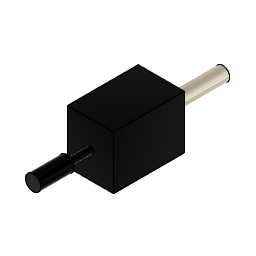
Large Solenoid Triggerable v13 (Autodesk Fusion 360 archive; units mm, degrees)
design "Self-retaining (two-way) Electromagnet DC 12V Push-pull Solenoid"
Autodesk Fusion 360 part; units mm, degrees
sketch "Sketch1" plane through (0, 0, 0) normal (0, 1, 0) x (1, 0, 0)
  line L0 (7.45, -8.575) -> (-7.45, -8.575)
  line L1 (-7.45, -8.575) -> (-7.45, 8.575)
  line L2 (-7.45, 8.575) -> (7.45, 8.575)
  line L3 (7.45, 8.575) -> (7.45, -8.575)
  line L4 (7.45, -8.575) -> (-7.45, 8.575) construction
  line L5 (-7.45, -8.575) -> (7.45, 8.575) construction
  circle A0 centre (0, 0) radius 1
  circle A1 centre (0, 0) radius 1.1
  dimension "d1" = 14.9
  dimension "d2" = 17.15
  dimension "d5" = 2.2
  dimension "d6" = 2
  constraint horizontal L0
  constraint perpendicular L0 L1
  constraint parallel L0 L2
  constraint parallel L1 L3
  constraint coincident L4 A0.centre
  constraint coincident L5 A0.centre
  constraint coincident A0.centre A1.centre
  measures "d1" distance of L1.end L2.end
  measures "d2" distance of L0.end L1.end
  measures "d5" diameter of A1
  measures "d6" diameter of A0
extrude "Extrude1" add sketch "Sketch1" along normal mid plane 22.85 contours L0 L1 L2 L3 makes body 1
extrude "Extrude2" add sketch "Sketch1" along normal blind 42.7 and the other way blind 18.5 from surface at -11.425 separate body contours A0 makes body 2
sketch "Sketch2" plane through (0, -29.925, 0) normal (0, -1, 0) x (1, 0, 0)
  circle A0 centre (0, 0) radius 1
  circle A1 centre (0, 0) radius 2.5
  dimension "d11" = 5
  constraint concentric A0 A1
  measures "d11" diameter of A1
extrude "Extrude3" add sketch "Sketch2" against normal blind 10.78 bodies 1 2
sketch "Sketch3" plane through (0, 31.275, 0) normal (0, 1, 0) x (-1, 0, 0)
  circle A0 centre (0, 0) radius 1
  circle A1 centre (0, 0) radius 2.25
  dimension "d15" = 4.5
  constraint concentric A0 A1
  measures "d15" diameter of A1
extrude "Extrude4" add sketch "Sketch3" against normal blind 14.5 bodies 2
copy_body "Body->Comp1" bodies 1 removing the originals makes body 3 in component "Body"
copy_body "Body->Comp2" bodies 2 removing the originals makes body 4 in component "Rod"
component "Body" placed x (1, 0, 0) y (0, 1, 0) z (0, 0, 1) at (0, 0, 0)
component "Rod" placed x (1, 0, 0) y (0, 1, 0) z (0, 0, 1) at (0, 0, 0)
equation "d5 = d6 + 0.2 mm"

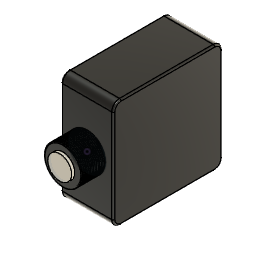
design "Tycon Circuit Breaker"
Autodesk Fusion 360 part; units mm, degrees
sketch "Sketch1" plane through (0, 0, 0) normal (0, 1, 0) x (1, 0, 0)
  line L0 (8.375, 17.45) -> (-8.375, 17.45)
  line L1 (-8.375, 17.45) -> (-8.375, -17.45)
  line L2 (-8.375, -17.45) -> (8.375, -17.45)
  line L3 (8.375, -17.45) -> (8.375, 17.45)
  line L4 (8.375, 17.45) -> (-8.375, -17.45) construction
  line L5 (-8.375, 17.45) -> (8.375, -17.45) construction
  dimension "d1" = 16.75
  dimension "d2" = 34.9
  constraint horizontal L0
  constraint perpendicular L0 L1
  constraint parallel L0 L2
  constraint parallel L1 L3
  constraint coincident L4 origin
  constraint coincident L5 origin
  measures "d1" distance of L1.end L2.end
  measures "d2" distance of L0.end L1.end
extrude "Extrude1" add sketch "Sketch1" along normal blind 35
sketch "Sketch2" plane through (0, 0, 0) normal (0, 1, 0) x (1, 0, 0)
  circle A0 centre (0, 0) radius 5.9
  dimension "d5" = 11.8
  constraint coincident A0.centre origin
  measures "d5" diameter of A0
extrude "Extrude2" add sketch "Sketch2" against normal blind 7.8
thread "Thread1" "ANSI Metric M Profile 12.0 M12x0.5 6g" major diameter 11.927 minor diameter 11.348 pitch 0.5 angle 60 modelled right hand crest width 0.0671 on face at (5.8707, -5.2, 0.5875) crest through (5.9635, 0.125, 0)
sketch "Sketch3" plane through (0, -7.8, 0) normal (0, -1, 0) x (1, 0, 0)
  spline S0 degree 3 poles (-5.3809, 1.8001) (-5.6333, 1.1023) (-5.7464, 0.3618) (-5.6834, -1.1281) (-5.5052, -1.863) (-4.8754, -3.2301) (-4.4274, -3.8481) (-3.3155, -4.8833) (-2.6605, -5.2886) (-1.4445, -5.7466) (-0.9193, -5.8662) (0.1522, -5.9611) (0.6936, -5.935) (1.2242, -5.8365) knots 0 0 0 0 0.222617 0.222617 0.447285 0.447285 0.674004 0.674004 0.902773 0.902773 1.063493 1.063493 1.22522 1.22522 1.22522 1.22522
  arc A0 (1.2242, -5.8365) -> (5.1726, -2.9678) centre (0, 0) ccw
  spline S1 degree 3 poles (5.1726, -2.9678) (5.5416, -2.2887) (5.7751, -1.5443) (5.9415, -0.0146) (5.8755, 0.7557) (5.4526, 2.2206) (5.1023, 2.9019) (4.1636, 4.0856) (3.5863, 4.5783) (2.4768, 5.2003) (1.9907, 5.3918) (0.9834, 5.6372) (0.4671, 5.6908) (-0.0492, 5.6738) knots 0 0 0 0 0.23188 0.23188 0.461709 0.461709 0.689485 0.689485 0.915208 0.915208 1.071357 1.071357 1.226496 1.226496 1.226496 1.226496
  arc A1 (-0.0492, 5.6738) -> (-5.3809, 1.8001) centre (0, 0) ccw
  circle A2 centre (0, 0) radius 3.825
  dimension "d8" = 7.65
  constraint concentric A0 A2
  measures "d8" diameter of A2
extrude "Extrude3" add sketch "Sketch3" along normal blind 1 contours A2
fillet "Fillet1" radius 2.5 4 edges at (0, 0, 17.45) (0, 35, 17.45) (0, 35, -17.45) (0, 0, -17.45)
fillet "Fillet1" radius 0.5 8 edges at (-8.375, 17.5, 17.45) (8.375, 17.5, 17.45) (8.375, 17.5, -17.45) (-8.375, 17.5, -17.45) (8.375, 0, 0) (-8.375, 0, 0) (-8.375, 35, 0) (8.375, 35, 0)
